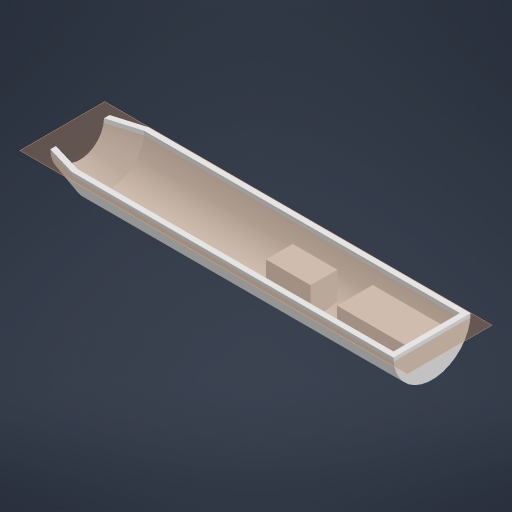
# Autodesk Inventor part: Half bottom
Saved by Autodesk Inventor 2023 (Build 270158000, 158)
## iProperties
Created: 2023-12-06
Part Number: Half bottom
Material: Generic
Document SubType Name: Modeling
Designer: Andi
Density: 1 g/cm^3
Appearance: Default
Author: Andi
Autodesk Inventor part; units mm, degrees
ref_plane "YZ Plane" through (0, 0, 0) normal (1, 0, 0) x (0, 1, 0)
ref_plane "XY Plane" through (0, 0, 0) normal (0, 0, 1) x (1, 0, 0)
sketch "Sketch1" plane through (0, 0, 0) normal (0, 1, 0) x (-1, 0, 0)
  line L0 (90, -21.5644) -> (-90, -21.5644)
  line L1 (-90, -21.5644) -> (-90, 0)
  line L2 (-90, 18.4356) -> (90, 18.4356) construction
  line L3 (90, -21.5644) -> (106.8856, -16.5644)
  line L4 (162.8256, 0) -> (106.8856, 13.4356) construction
  line L5 (106.8856, -16.5644) -> (106.8856, -13.4356)
  line L6 (106.8856, -16.5644) -> (162.8256, 0) construction
  line L7 (106.8856, 13.4356) -> (90, 18.4356) construction
  line L8 (162.8256, 0) -> (-90, 0)
  line L9 (-87, -18.5644) -> (89.5652, -18.5644)
  line L10 (89.5652, -18.5644) -> (106.8856, -13.4356)
  line L11 (-90, 0) -> (-87, 0)
  line L12 (-87, 0) -> (-87, -18.5644)
  line L13 (106.8856, 0) -> (106.8856, 13.4356) construction
  line L14 (-90, 0) -> (-90, 18.4356) construction
  line L15 (106.8856, -13.4356) -> (106.8856, 0) construction
  point P0 (0, 0)
  point P1 (108.6603, 0)
  point P2 (-87, 0)
  dimension "d0" = 180
  dimension "d1" = 40
  dimension "d2" = 3
  dimension "d3" = 3
  dimension "d5" = 30
  dimension "d6" = 90
  dimension "d7" = 30
  dimension "d9" = 3
  constraints: 32 end point, 5 perpendicular, 3 equal length, 3 horizontal alignment, 3 vertical, 1 collinear, 1 horizontal, 1 parallel
  measures "d0" distance of L2.start L2.end
  measures "d1" distance of L0.end L2.start
  measures "d2" distance between parallel lines of L9 L0
  measures "d3" distance between parallel lines of L12 L1
  measures "d5" angle of L4 L6
  measures "d6" distance from line of point (0, 0) L1
  measures "d7" distance of L4.end L3.end
  measures "d9" distance between parallel lines of L10 L3
revolve "Revolution1" add sketch "Sketch1" angle 180 about axis through (-162.8256, 0, 0) along (-1, 0, 0)
ref_plane "Work Plane1" through (0, -2, 0) normal (0, 1, 0) x (-1, 0, 0)
sketch "Sketch2" plane through (0, -2, 0) normal (0, 1, 0) x (-1, 0, 0)
  line L0 (-47, -9.8426) -> (-87, -9.8426)
  line L1 (-87, -9.8426) -> (-87, 10.1574)
  line L2 (-87, 10.1574) -> (-47, 10.1574)
  line L3 (-47, 10.1574) -> (-47, -9.8426)
  line L4 (-87, -18.5644) -> (-87, 18.5644) construction
  line L5 (-87, -18.5644) -> (-87, 18.5644) construction
  line L6 (-4.7327, -7.3426) -> (-29.7327, -7.3426)
  line L7 (-29.7327, -7.3426) -> (-29.7327, 7.6574)
  line L8 (-29.7327, 7.6574) -> (-4.7327, 7.6574)
  line L9 (-4.7327, 7.6574) -> (-4.7327, -7.3426)
  point P0 (0, 0)
  point P1 (-87, 0)
  point P2 (-47, 0.1574)
  point P3 (-29.7327, 0.1574)
  point P4 (-87, 0)
  point P5 (-87, 0)
  point P6 (-87, 0)
  dimension "d18" = 40
  dimension "d19" = 20
  dimension "d20" = 25
  dimension "d21" = 15
  constraints: 16 end point, 4 parallel, 4 point on line, 3 midpoint, 2 horizontal, 2 perpendicular, 1 horizontal alignment
  measures "d18" distance of L0.start L0.end
  measures "d19" distance of L2.end L0.start
  measures "d20" distance of L6.start L6.end
  measures "d21" distance of L8.end L6.start
extrude "Extrusion1" add sketch "Sketch2" against normal up to surface round surface about axis through (-1.2826, 0, 0) along (-1, 0, 0) radius 18.5644 far side no
equation "\"d3\" = d2"
equation "\"d9\" = d2"
body "Solid1"
